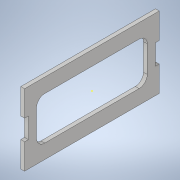
# Autodesk Inventor part: open_case
Saved by Autodesk Inventor 2020 (Build 240168000, 168)
## iProperties
Created: 2019-12-18
Part Number: open_case
Material: Generic
Document SubType Name: Modeling
Designer: fabfarm
Density: 1 g/cm^3
Appearance: Default
Author: fabfarm
Autodesk Inventor part; units mm, degrees
ref_plane "YZ Plane" through (0, 0, 0) normal (1, 0, 0) x (0, 1, 0)
ref_plane "XZ Plane" through (0, 0, 0) normal (0, 1, 0) x (-1, 0, 0)
ref_plane "XY Plane" through (0, 0, 0) normal (0, 0, 1) x (1, 0, 0)
sketch "Sketch1" plane through (0, 0, 0) normal (1, 0, 0) x (0, 1, 0)
  line L0 (-175, -330) -> (175, -330)
  line L1 (175, -330) -> (175, 330)
  line L2 (175, 330) -> (-175, 330)
  line L3 (-175, 330) -> (-175, -330)
  line L4 (-175, -330) -> (175, 330) construction
  line L5 (175, -330) -> (-175, 330) construction
  point P0 (0, 0)
  dimension "d0" = 660
  dimension "d1" = 350
  constraints: 12 end point, 2 midpoint, 2 parallel, 1 horizontal, 1 perpendicular
  measures "d0" distance of L0.end L1.end
  measures "d1" distance of L0.start L0.end
extrude "Extrusion1" add sketch "Sketch1" along normal blind 18.55
sketch "Sketch2" plane through (18.55, 0, 0) normal (1, 0, 0) x (0, 0, -1)
  line L0 (-330, 175) -> (-330, -175) projected
  line L1 (-330, -50) -> (-311.45, -50)
  line L2 (-311.45, -50) -> (-311.45, 50)
  line L3 (-311.45, 50) -> (-330, 50)
  line L4 (-330, 50) -> (-330, -50)
  line L5 (330, 175) -> (-330, 175) projected
  point P0 (0, 0)
  dimension "d5" = 18.55
  dimension "d6" = 100
  dimension "d20" = 125
  constraints: 8 end point, 2 parallel, 1 horizontal, 1 perpendicular, 1 point on line
  measures "d5" distance of L2.end L3.end
  measures "d6" distance of L1.end L2.end
  measures "d20" distance between parallel lines of L5 L3
extrude "Extrusion2" cut sketch "Sketch2" against normal blind 18.55
mirror "Mirror1" about plane through (0, 0, 0) normal (0, 0, 1) of "Extrusion2"
sketch "Sketch3" plane through (18.55, 0, 0) normal (1, 0, 0) x (0, 0, -1)
  line L0 (231.45, -105) -> (-231.45, -105)
  line L1 (-271.45, -65) -> (-271.45, 65)
  line L2 (-231.45, 105) -> (231.45, 105)
  line L3 (271.45, 65) -> (271.45, -65)
  line L4 (271.45, -105) -> (-271.45, 105) construction
  line L5 (-271.45, -105) -> (271.45, 105) construction
  line L6 (-330, 50) -> (-311.45, 50) projected
  arc A0 (-231.45, 105) -> (-271.45, 65) centre (-231.45, 65) ccw
  arc A1 (-271.45, -65) -> (-231.45, -105) centre (-231.45, -65) ccw
  arc A2 (271.45, 65) -> (231.45, 105) centre (231.45, 65) ccw
  arc A3 (231.45, -105) -> (271.45, -65) centre (231.45, -65) ccw
  line L7 (-330, -50) -> (-330, -175) projected
  line L8 (-311.45, 50) -> (-311.45, -50) projected
  line L9 (330, 175) -> (-330, 175) projected
  point P0 (0, 0)
  dimension "d23" = 40
  dimension "d24" = 40
  dimension "d25" = 70
  constraints: 12 end point, 8 point on circle, 8 point on line, 8 tangent, 4 centre point, 3 equal radius, 2 midpoint, 2 parallel, 1 horizontal, 1 perpendicular
  measures "d23" distance between parallel lines of L8 L1
  measures "d24" radius of A0
  measures "d25" distance between parallel lines of L9 L2
extrude "Extrusion3" cut sketch "Sketch3" against normal blind 18.55
sketch "Esquisse4" plane through (18.55, 0, 0) normal (1, 0, 0) x (0, 0, -1)
  point P0 (0, 0)
body "Solid1"
